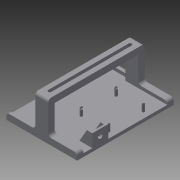
# Autodesk Inventor part: new_base
Saved by Autodesk Inventor 2015 (Build 190159000, 159)
## iProperties
Created: 2014-12-16
Part Number: new_base
Material: Generic
Document SubType Name: Modeling
Designer: Rene
Density: 1 g/cm^3
Appearance: Default
Author: Rene
Autodesk Inventor part; units mm, degrees
ref_plane "YZ Plane" through (0, 0, 0) normal (1, 0, 0) x (0, 1, 0)
ref_plane "XZ Plane" through (0, 0, 0) normal (0, 1, 0) x (-1, 0, 0)
ref_plane "XY Plane" through (0, 0, 0) normal (0, 0, 1) x (1, 0, 0)
sketch "Sketch1" plane through (0, 0, 0) normal (0, 1, 0) x (-1, 0, 0)
  line L0 (139.7, 190.5) -> (0, 190.5)
  line L1 (0, 190.5) -> (0, 0)
  line L2 (0, 0) -> (139.7, 0)
  line L3 (139.7, 0) -> (139.7, 190.5)
  dimension "d0" = 190.5
  dimension "d1" = 139.7
  constraints: 8 end point, 2 parallel, 1 horizontal, 1 perpendicular
  measures "d0" distance of L2.end L0.start
  measures "d1" distance of L0.start L0.end
extrude "Extrusion1" add sketch "Sketch1" along normal blind 6.35
sketch "Sketch2" plane through (0, 6.35, 0) normal (0, 1, 0) x (1, 0, 0)
  line L0 (0, -190.5) -> (0, 0) projected
  line L1 (-139.7, 0) -> (0, 0)
  line L2 (0, 0) -> (0, -12.7)
  line L3 (0, -12.7) -> (-139.7, -12.7)
  line L4 (-139.7, -12.7) -> (-139.7, 0)
  line L5 (-139.7, -190.5) -> (0, -190.5)
  line L6 (0, -190.5) -> (0, -177.8)
  line L7 (0, -177.8) -> (-139.7, -177.8)
  line L8 (-139.7, -177.8) -> (-139.7, -190.5)
  dimension "d4" = 12.7
  dimension "d5" = 12.7
  constraints: 16 end point, 4 parallel, 2 horizontal, 2 perpendicular, 2 point on line
  measures "d4" distance between parallel lines of L3 L1
  measures "d5" distance between parallel lines of L5 L7
extrude "Extrusion2" add sketch "Sketch2" along normal blind 6.35
sketch "Sketch3" plane through (0, 12.7, 0) normal (0, 1, 0) x (1, 0, 0)
  line L0 (0, 0) -> (-139.7, 0) projected
  line L1 (-139.7, -12.7) -> (0, -12.7) projected
  line L2 (-82.55, 0) -> (-57.15, 0)
  line L3 (-57.15, 0) -> (-57.15, -12.7)
  line L4 (-57.15, -12.7) -> (-82.55, -12.7)
  line L5 (-82.55, -12.7) -> (-82.55, 0)
  line L6 (-139.7, 0) -> (-139.7, -12.7) projected
  line L7 (0, -12.7) -> (0, 0) projected
  line L8 (0, -177.8) -> (-139.7, -177.8) projected
  line L9 (-139.7, -190.5) -> (0, -190.5) projected
  line L10 (-82.55, -177.8) -> (-57.15, -177.8)
  line L11 (-57.15, -177.8) -> (-57.15, -190.5)
  line L12 (-57.15, -190.5) -> (-82.55, -190.5)
  line L13 (-82.55, -190.5) -> (-82.55, -177.8)
  line L14 (-139.7, -177.8) -> (-139.7, -190.5) projected
  line L15 (0, -190.5) -> (0, -177.8) projected
  dimension "d8" = 139.7
  dimension "d9" = 57.15
  dimension "d10" = 57.15
  dimension "d11" = 57.15
  dimension "d12" = 57.15
  constraints: 16 end point, 4 parallel, 4 point on line, 2 horizontal, 2 perpendicular
  measures "d8" distance of L0.start L0.end
  measures "d9" distance between parallel lines of L6 L5
  measures "d10" distance between parallel lines of L7 L3
  measures "d11" distance between parallel lines of L14 L13
  measures "d12" distance between parallel lines of L15 L11
extrude "Extrusion3" add sketch "Sketch3" along normal blind 63.5 contours L3 L1 L5 L0 | L11 L9 L13 L8
sketch "Sketch4" plane through (0, 6.35, 177.8) normal (0, 0, -1) x (-1, 0, 0)
  line L0 (82.55, 6.35) -> (82.55, 69.85) projected
  line L1 (57.15, 69.85) -> (82.55, 69.85)
  line L2 (82.55, 69.85) -> (82.55, 57.15)
  line L3 (82.55, 57.15) -> (57.15, 57.15)
  line L4 (57.15, 57.15) -> (57.15, 69.85)
  point P0 (0, -6.35)
  dimension "d15" = 12.7
  constraints: 8 end point, 2 parallel, 1 horizontal, 1 perpendicular, 1 point on line
  measures "d15" distance between parallel lines of L3 L1
extrude "Extrusion4" add sketch "Sketch4" along normal blind 177.8
sketch "Sketch5" plane through (0, 76.2, 0) normal (0, 1, 0) x (1, 0, 0)
  line L0 (-66.675, -12.7) -> (-73.025, -12.7)
  line L1 (-73.025, -12.7) -> (-73.025, -177.8)
  line L2 (-73.025, -177.8) -> (-66.675, -177.8)
  line L3 (-66.675, -177.8) -> (-66.675, -12.7)
  line L4 (-57.15, 0) -> (-82.55, 0) projected
  line L5 (-57.15, -190.5) -> (-57.15, 0) projected
  line L6 (-82.55, 0) -> (-82.55, -190.5) projected
  line L7 (-82.55, -190.5) -> (-57.15, -190.5) projected
  point P0 (0, 0)
  dimension "d18" = 12.7
  dimension "d19" = 6.35
  dimension "d20" = 9.525
  dimension "d21" = 9.525
  dimension "d22" = 12.7
  constraints: 8 end point, 2 parallel, 1 horizontal, 1 perpendicular
  measures "d18" distance between parallel lines of L4 L0
  measures "d19" distance of L1.end L2.end
  measures "d20" distance between parallel lines of L5 L3
  measures "d21" distance between parallel lines of L6 L1
  measures "d22" distance between parallel lines of L2 L7
extrude "Extrusion5" cut sketch "Sketch5" against normal blind 25.4 contours L3 L2 L1 L0
fillet "Fillet1" radius 6.35 10 edges at (-139.7, 12.7, 6.35) (-82.55, 12.7, 6.35) (-139.7, 12.7, 184.15) (-82.55, 12.7, 184.15) (-57.15, 12.7, 184.15) (0, 12.7, 184.15) (0, 12.7, 6.35) (-57.15, 12.7, 6.35) (-69.85, 76.2, 0) (-69.85, 76.2, 190.5)
fillet "Fillet2" radius 3.175 4 edges at (-73.025, 69.85, 12.7) (-73.025, 69.85, 177.8) (-66.675, 69.85, 177.8) (-66.675, 69.85, 12.7)
sketch "Sketch7" plane through (0, 6.35, 0) normal (0, 1, 0) x (1, 0, 0)
  line L0 (0, -177.8) -> (0, -12.7) projected
  line L1 (0, -154.1443) -> (-25.4, -154.1443)
  line L2 (-25.4, -154.1443) -> (-25.4, -128.7443)
  line L3 (-25.4, -128.7443) -> (0, -128.7443)
  line L4 (0, -128.7443) -> (0, -154.1443)
  point P0 (0, 0)
  dimension "d41" = 25.4
  dimension "d42" = 25.4
  constraints: 8 end point, 2 parallel, 1 horizontal, 1 perpendicular, 1 point on line
  measures "d41" distance of L1.end L2.end
  measures "d42" distance of L2.end L3.end
extrude "Extrusion7" add sketch "Sketch7" along normal blind 25.4
sketch "Sketch9" plane through (0, 31.75, 0) normal (0, 1, 0) x (1, 0, 0)
  line L0 (-25.4, -133.8243) -> (-3.81, -133.8243)
  line L1 (-3.81, -133.8243) -> (-3.81, -149.0643)
  line L2 (-3.81, -149.0643) -> (-25.4, -149.0643)
  line L3 (-25.4, -149.0643) -> (-25.4, -133.8243)
  line L4 (-25.4, -128.7443) -> (-25.4, -154.1443) projected
  line L5 (-25.4, -154.1443) -> (0, -154.1443) projected
  line L6 (0, -128.7443) -> (-25.4, -128.7443) projected
  line L7 (0, -154.1443) -> (0, -128.7443) projected
  point P0 (0, 0)
  dimension "d46" = 0
  dimension "d47" = 5.08
  dimension "d48" = 5.08
  dimension "d49" = 3.81
  constraints: 8 end point, 2 parallel, 1 horizontal, 1 perpendicular
  measures "d46" distance between parallel lines of L4 L3
  measures "d47" distance between parallel lines of L5 L2
  measures "d48" distance between parallel lines of L6 L0
  measures "d49" distance between parallel lines of L7 L1
extrude "Extrusion8" cut sketch "Sketch9" against normal blind 25.4 contours L0 L1 L2 L3
sketch "Sketch10" plane through (0, 0, 190.5) normal (1, 0, 0) x (0, 0, -1)
  circle A0 centre (49.0557, 19.05) radius 5.588
  line L0 (36.3557, 31.75) -> (61.7557, 31.75) projected
  line L1 (36.3557, 6.35) -> (36.3557, 31.75) projected
  point P0 (190.5, 0)
  dimension "d52" = 12.7
  dimension "d53" = 12.7
  dimension "d54" = 11.176
  constraints: 1 centre point
  measures "d52" distance from line of L0 A0.centre
  measures "d53" distance from line of L1 A0.centre
  measures "d54" diameter of A0
extrude "Extrusion9" cut sketch "Sketch10" against normal blind 25.4
sketch "Sketch11" plane through (0, 6.35, 128.7443) normal (0, 0, -1) x (-1, 0, 0)
  line L0 (25.4, 0) -> (10.7353, 25.4)
  line L1 (0, 25.4) -> (25.4, 25.4) projected
  line L2 (25.4, 0) -> (0, 0) projected
  line L3 (10.7353, 25.4) -> (25.4, 25.4)
  line L4 (25.4, 25.4) -> (25.4, 0)
  line L5 (25.4, 0) -> (25.4, 25.4) projected
  point P0 (0, -6.35)
  dimension "d57" = 60
  constraints: 6 end point, 1 collinear, 1 horizontal, 1 point on line
  measures "d57" angle of L2 L0
extrude "Extrusion10" cut sketch "Sketch11" against normal blind 25.4
sketch "Sketch12" plane through (0, 6.35, 0) normal (0, 1, 0) x (1, 0, 0)
  circle A0 centre (-12.7, -116.0443) radius 2.4765
  line L0 (0, -128.7443) -> (0, -12.7) projected
  line L1 (-25.4, -128.7443) -> (0, -128.7443) projected
  circle A1 centre (-12.7, -47.2103) radius 2.4765
  circle A2 centre (-66.294, -116.0443) radius 2.4765
  circle A3 centre (-66.294, -47.2103) radius 2.4765
  point P0 (0, 0)
  dimension "d60" = 12.7
  dimension "d61" = 12.7
  dimension "d62" = 68.834
  dimension "d63" = 4.953
  dimension "d64" = 4.953
  dimension "d65" = 4.953
  dimension "d66" = 53.594
  dimension "d67" = 4.953
  dimension "d68" = 53.594
  dimension "d69" = 68.834
  constraints: 4 centre point
  measures "d60" distance from line of L0 A0.centre
  measures "d61" distance from line of L1 A0.centre
  measures "d62" distance of A0.centre A1.centre
  measures "d63" diameter of A1
  measures "d64" diameter of A0
  measures "d65" diameter of A2
  measures "d66" distance of A2.centre A0.centre
  measures "d67" diameter of A3
  measures "d68" distance of A1.centre A3.centre
  measures "d69" distance of A2.centre A3.centre
extrude "Extrusion11" add sketch "Sketch12" along normal blind 15.24
sketch "Sketch13" plane through (-12.7, 21.59, 116.0443) normal (0, 1, 0) x (1, 0, 0)
  circle A0 centre (0, 0) radius 0.889
  circle A1 centre (0, 0) radius 2.4765 projected
  circle A2 centre (-53.594, 0) radius 0.889
  circle A3 centre (-53.594, 0) radius 2.4765 projected
  circle A4 centre (0, 68.834) radius 0.889
  circle A5 centre (0, 68.834) radius 2.4765 projected
  circle A6 centre (-53.594, 68.834) radius 0.889
  circle A7 centre (-53.594, 68.834) radius 2.4765 projected
  point P0 (12.7, 116.0443)
  dimension "d72" = 1.778
  dimension "d73" = 0
  dimension "d74" = 0
  dimension "d75" = 0
  dimension "d76" = 0
  dimension "d77" = 1.778
  dimension "d78" = 1.778
  dimension "d79" = 0
  dimension "d80" = 0
  dimension "d81" = 1.778
  dimension "d82" = 0
  dimension "d83" = 0
  constraints: 4 centre point
  measures "d72" diameter of A0
  measures "d73" distance of A0.centre A1.centre
  measures "d74" distance of A1.centre A0.centre
  measures "d75" distance of A3.centre A2.centre
  measures "d76" distance of A2.centre A3.centre
  measures "d77" diameter of A2
  measures "d78" diameter of A4
  measures "d79" distance of A5.centre A4.centre
  measures "d80" distance of A5.centre A4.centre
  measures "d81" diameter of A6
  measures "d82" distance of A7.centre A6.centre
  measures "d83" distance of A7.centre A6.centre
extrude "Extrusion12" cut sketch "Sketch13" against normal blind 11.43 contours A0 | A2 | A4 | A6
sketch "Sketch17" plane through (-12.7, 21.59, 47.2103) normal (0, 1, 0) x (1, 0, 0)
  circle A0 centre (0, -68.834) radius 2.4765 projected
  circle A1 centre (-53.594, 0) radius 2.4765 projected
  line L0 (0, -71.3105) -> (-53.594, -71.3105)
  line L1 (-53.594, -71.3105) -> (-53.594, 2.4765)
  line L2 (-53.594, 2.4765) -> (0, 2.4765)
  line L3 (0, 2.4765) -> (0, -71.3105)
  point P0 (12.7, 47.2103)
  constraints: 8 end point, 2 parallel, 2 vertical alignment, 1 horizontal, 1 perpendicular, 2 other
extrude "Extrusion13" cut sketch "Sketch17" against normal blind 3.175 contours L0 L1 A1 L2 L3 A0 | A0 L3 | L1 A1 picked at (-0.3836, -69.5649) picked at (-53.0521, 0.7644)
sketch "Sketch18" plane through (0, 6.35, 154.1443) normal (0, 0, 1) x (1, 0, 0)
  line L0 (-10.7353, 25.4) -> (-25.4, 0) projected
  line L1 (0, 0) -> (-25.4, 0) projected
  line L2 (0, 0) -> (0, 25.4) projected
  line L3 (-10.7353, 25.4) -> (0, 25.4) projected
  point P0 (0, -6.35)
extrude "Extrusion14" add sketch "Sketch18" along normal blind 6.35
sketch "Sketch19" plane through (0, 31.75, 0) normal (0, 1, 0) x (1, 0, 0)
  line L0 (-10.7353, -133.8243) -> (-3.81, -133.8243) projected
  line L1 (0, -128.7443) -> (-10.7353, -128.7443) projected
  line L2 (-25.4, -160.4943) -> (-25.4, -149.0643) projected
  line L3 (-3.81, -133.8243) -> (-25.4, -133.8243)
  line L4 (-25.4, -133.8243) -> (-25.4, -155.4143)
  line L5 (-25.4, -155.4143) -> (-3.81, -155.4143)
  line L6 (-3.81, -155.4143) -> (-3.81, -133.8243)
  line L7 (0, -160.4943) -> (-10.7353, -160.4943) projected
  point P0 (0, 0)
  dimension "d99" = 5.08
  dimension "d100" = 5.08
  constraints: 8 end point, 2 parallel, 1 horizontal, 1 perpendicular, 1 point on line
  measures "d99" distance between parallel lines of L0 L1
  measures "d100" distance between parallel lines of L7 L5
extrude "Extrusion18" cut sketch "Sketch19" against normal blind 25.4
sketch "Sketch22" plane through (0, 0, 190.5) normal (1, 0, 0) x (0, 0, -1)
  line L0 (38.5018, 28.1122) -> (55.9606, 28.1122)
  line L1 (55.9606, 28.1122) -> (55.9606, 11.081)
  line L2 (55.9606, 11.081) -> (38.5018, 11.081)
  line L3 (38.5018, 11.081) -> (38.5018, 28.1122)
  point P0 (190.5, 0)
  constraints: 8 end point, 2 parallel, 1 horizontal, 1 perpendicular
extrude "Extrusion19" add sketch "Sketch22" against normal blind 3.81
sketch "Sketch24" plane through (0, 0, 190.5) normal (1, 0, 0) x (0, 0, -1)
  circle A0 centre (45.8807, 19.05) radius 4.6631
  line L0 (56.6757, 6.35) -> (35.0857, 6.35) projected
  line L1 (56.6757, 31.75) -> (56.6757, 6.35) projected
  line L2 (35.0857, 31.75) -> (35.0857, 6.35) projected
  point P0 (190.5, 0)
  dimension "d113" = 12.7
  dimension "d114" = 10.795
  dimension "d115" = 21.59
  constraints: 1 centre point
  measures "d113" distance from line of L0 A0.centre
  measures "d114" distance from line of L1 A0.centre
  measures "d115" distance between parallel lines of L1 L2
extrude "Extrusion20" cut sketch "Sketch24" against normal blind 3.81
sketch "Sketch31" plane through (0, 6.35, 0) normal (0, 1, 0) x (1, 0, 0)
  line L0 (-139.7, -190.5) -> (-139.7, 0) projected
  line L1 (-82.55, -190.5) -> (-82.55, -177.8) projected
  line L2 (-139.7, -6.35) -> (-82.55, -6.35)
  line L3 (-82.55, -6.35) -> (-82.55, -184.15)
  line L4 (-82.55, -184.15) -> (-139.7, -184.15)
  line L5 (-139.7, -184.15) -> (-139.7, -6.35)
  line L6 (-82.55, -190.5) -> (-57.15, -190.5) projected
  point P0 (0, 0)
  dimension "d139" = 57.15
  dimension "d140" = 177.8
  dimension "d141" = 6.35
  constraints: 8 end point, 2 parallel, 1 horizontal, 1 midpoint, 1 perpendicular, 1 point on line
  measures "d139" distance of L2.start L2.end
  measures "d140" distance of L2.end L3.end
  measures "d141" distance between parallel lines of L6 L4
extrude "Extrusion22" cut sketch "Sketch31" along normal blind 12.7
body "Solid1"
